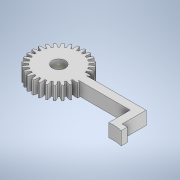
# Autodesk Inventor part: NewConceptArm free V2
Saved by Autodesk Inventor 2022 (Build 260153000, 153)
## iProperties
Created: 2022-02-25
Part Number: NewConceptArm free V2
Material: Generic
Document SubType Name: Modeling
Designer: Alexa
Density: 1 g/cm^3
Appearance: Default
Author: Alexa
Autodesk Inventor part; units mm, degrees
ref_plane "YZ Plane" through (0, 0, 0) normal (1, 0, 0) x (0, 1, 0)
ref_plane "XZ Plane" through (0, 0, 0) normal (0, 1, 0) x (-1, 0, 0)
ref_plane "XY Plane" through (0, 0, 0) normal (0, 0, 1) x (1, 0, 0)
sketch "Sketch1" plane through (0, 0, 0) normal (0, 1, 0) x (-1, 0, 0)
  circle A0 centre (0, 0) radius 8
  circle A1 centre (0, 0) radius 2
  line L0 (7.9113, 0.5933) -> (7.9113, -0.6067)
  line L1 (9.9113, -0.2567) -> (9.9113, 0.2433)
  line L2 (7.6237, -0.0067) -> (9.0479, -0.0067) construction
  arc A2 (9.9113, 0.2433) -> (7.9113, 0.5933) centre (8.1555, -3.9001) ccw construction
  arc A3 (7.9113, -0.6067) -> (9.9113, -0.2567) centre (8.1555, 3.8866) ccw construction
  arc A4 (9.9113, 0.2433) -> (7.9113, 0.5933) centre (8.1555, -3.9001) ccw construction
  arc A5 (9.9113, 0.2433) -> (7.9777, 0.5964) centre (8.1555, -3.9001) ccw
  arc A6 (7.9767, -0.6098) -> (9.9113, -0.2567) centre (8.1555, 3.8866) ccw
  line L3 (9.4, 0) -> (9.4, -0.4379)
  line L4 (9.4, 0) -> (9.4, 0.4244)
  arc A7 (5.296, -1.8919) -> (5.296, 1.8784) centre (4.6281, -0.0067) ccw
  circle A8 centre (0, 0) radius 8
  dimension "d0" = 16
  dimension "d1" = 4
  dimension "d2" = 0.25
  dimension "d3" = 0.25
  dimension "d4" = 0.6
  dimension "d7" = 1.2
  dimension "d8" = 4.5
  dimension "d10" = 2
  constraints: 18 point on circle, 10 end point, 9 centre point, 4 concentric, 3 coincident, 2 vertical, 1 horizontal, 1 parallel, 1 point on line
  measures "d0" diameter of A0
  measures "d1" diameter of A1
  measures "d2" distance from line of L1.start L2
  measures "d3" distance from line of L1.end L2
  measures "d4" distance from line of L0.start L2
  measures "d7" distance of L0.end L0.start
  measures "d8" radius of A3
  measures "d10" radius of A7
extrude "Extrusion1" add sketch "Sketch1" along normal blind 5
pattern_circular "Circular Pattern1" count 28 over 360 about axis through (0, 0, 0) along (0, 1, 0) of "Extrusion1"
sketch "Sketch8" plane through (0, 5, 0) normal (0, 1, 0) x (1, 0, 0)
  circle A0 centre (0, 0) radius 2.5
  circle A1 centre (0, 0) radius 2
  dimension "d49" = 5
  dimension "d50" = 4
  constraints: 2 centre point, 2 coincident
  measures "d49" diameter of A0
  measures "d50" diameter of A1
extrude "Extrusion6" cut sketch "Sketch8" against normal blind 13.8125
sketch "Sketch9" plane through (0, 5, 0) normal (0, 1, 0) x (1, 0, 0)
  circle A0 centre (0, 0) radius 2.5 projected
  line L0 (0, 0) -> (30, 0)
  line L1 (30, 0) -> (30, -18)
  line L2 (30, -18) -> (0, -18)
  line L3 (0, -18) -> (0, 0)
  circle A1 centre (0, 0) radius 9.5
  circle A2 centre (0, -18) radius 9.5
  line L4 (30, -9) -> (0, -9)
  circle A3 centre (30, -9) radius 2.5
  line L5 (30, 0) -> (5, 0)
  line L6 (5, 0) -> (5, -1.5)
  line L7 (5, -1.5) -> (30, -1.5)
  line L8 (30, -1.5) -> (30, 0)
  line L9 (5, 0) -> (30, 0)
  line L10 (30, 0) -> (30, 1.5)
  line L11 (30, 1.5) -> (5, 1.5)
  line L12 (5, 1.5) -> (5, 0)
  line L13 (30, 1.5) -> (31.5, 1.5)
  line L14 (31.5, 1.5) -> (31.5, -7.5)
  line L15 (31.5, -7.5) -> (30, -7.5)
  line L16 (30, -7.5) -> (30, 1.5)
  line L17 (30, 1.5) -> (28.5, 1.5)
  line L18 (28.5, 1.5) -> (28.5, -7.5)
  line L19 (28.5, -7.5) -> (30, -7.5)
  line L20 (30, -7.5) -> (30, 1.5)
  circle A4 centre (30, -9) radius 1.5
  line L21 (27.5, -9) -> (32.5, -9)
  line L22 (32.5, -9) -> (32.5, -8.5)
  line L23 (32.5, -8.5) -> (27.5, -8.5)
  line L24 (27.5, -8.5) -> (27.5, -9)
  line L25 (28.5, -7.5) -> (27.5, -8.5)
  line L26 (31.5, -7.5) -> (32.5, -8.5)
  line L27 (27.5, -8.5) -> (28.5, -8.5)
  line L28 (32.5, -8.5) -> (31.5, -8.5)
  line L29 (28.5, -7.5) -> (29, -7.5)
  line L30 (31.5, -7.5) -> (31, -7.5)
  line L31 (31, -7.5) -> (31.5, -8.5)
  line L32 (29, -7.5) -> (28.5, -8.5)
  line L33 (5, 1.5) -> (12.096, 1.5)
  line L34 (12.096, 1.5) -> (12.096, -1.5)
  line L35 (12.096, -1.5) -> (5, -1.5)
  line L36 (5, -1.5) -> (5, 1.5)
  dimension "d57" = 5
  dimension "d53" = 30
  dimension "d54" = 18
  dimension "d55" = 19
  dimension "d56" = 19
  dimension "d58" = 25
  dimension "d59" = 1.5
  dimension "d60" = 1.5
  dimension "d61" = 1.5
  dimension "d62" = 9
  dimension "d63" = 1.5
  dimension "d64" = 3
  dimension "d65" = 5
  dimension "d66" = 0.5
  dimension "d67" = 0.5
  dimension "d68" = 0.5
  constraints: 74 end point, 14 parallel, 10 point on line, 7 horizontal, 7 perpendicular, 4 coincident, 3 centre point, 2 midpoint, 1 horizontal alignment, 2 other
  measures "d53" distance of L1.end L2.end
  measures "d54" distance of L0.end L1.end
  measures "d55" diameter of A1
  measures "d56" diameter of A2
  measures "d58" distance of L7.end L6.end
  measures "d59" distance of L6.end L5.end
  measures "d60" distance of L10.end L9.end
  measures "d61" distance of L14.end L15.end
  measures "d62" distance of L13.end L14.end
  measures "d63" distance of L19.end L18.end
  measures "d64" diameter of A4
  measures "d65" distance of L23.end L22.end
  measures "d66" distance of L22.end L21.end
  measures "d67" distance of L18.end L29.end
  measures "d68" distance of L14.end L30.end
extrude "Extrusion7" cut sketch "Sketch9" against normal blind 5 contours L12 L11 A1 L0 | L0 A1 L7 L6 | A1 L11 L34 L0 | L0 L34 L7 A1
sketch "Sketch10" plane through (0, 5, 0) normal (0, 1, 0) x (1, 0, 0)
  circle A0 centre (0, 0) radius 2.5 projected
  line L0 (0, 0) -> (30, 0)
  line L1 (30, 0) -> (30, -9)
  line L2 (30, -9) -> (0, -9)
  line L3 (0, -9) -> (0, 0)
  line L4 (5, 1.5) -> (30, 1.5)
  line L5 (30, 1.5) -> (30, -1.5)
  line L6 (30, -1.5) -> (5, -1.5)
  line L7 (5, -1.5) -> (5, 1.5)
  line L8 (31.5, 1.5) -> (28.5, 1.5)
  line L9 (28.5, 1.5) -> (28.5, -7.5)
  line L10 (28.5, -7.5) -> (31.5, -7.5)
  line L11 (31.5, -7.5) -> (31.5, 1.5)
  circle A1 centre (30, -9) radius 1.5
  circle A2 centre (30, -9) radius 2.5
  line L12 (27.5, -9) -> (32.4495, -9)
  line L13 (32.4495, -9) -> (32.4495, -8.5)
  line L14 (27.5, -8.5) -> (27.5, -9)
  line L15 (27.5, -9) -> (32.5, -9)
  line L16 (32.5, -9) -> (32.5, -8.5)
  line L17 (32.5, -8.5) -> (27.5, -8.5)
  line L18 (27.5, -8.5) -> (27.5, -9)
  line L19 (28.5, -7.5) -> (27.5, -8.5)
  line L20 (31.5, -7.5) -> (32.5, -8.5)
  line L21 (28.5, -7.5) -> (29, -7.5)
  line L22 (31.5, -7.5) -> (31, -7.5)
  line L23 (29, -7.5) -> (28.5, -8.5)
  line L24 (31, -7.5) -> (31.5, -8.5)
  point P0 (28.5, -1.5)
  point P1 (28.5, -7)
  point P2 (27.5505, -8.5)
  point P3 (28.5858, -8.5)
  point P4 (31.4142, -8.5)
  point P5 (31.5, -7)
  dimension "d71" = 30
  dimension "d72" = 9
  dimension "d73" = 3
  dimension "d74" = 3
  dimension "d75" = 9
  dimension "d76" = 3
  dimension "d77" = 5
  dimension "d78" = 0.5
  dimension "d79" = 5
  dimension "d80" = 0.5
  dimension "d81" = 0.5
  constraints: 50 end point, 9 parallel, 7 point on line, 6 perpendicular, 5 horizontal, 2 centre point, 2 coincident, 2 point on circle
  measures "d71" distance of L1.end L2.end
  measures "d72" distance of L0.end L1.end
  measures "d73" distance of L4.end L5.end
  measures "d74" distance of L10.end L9.end
  measures "d75" distance of L9.end L8.end
  measures "d76" diameter of A1
  measures "d77" diameter of A2
  measures "d78" distance of L13.end L12.end
  measures "d79" distance of L17.end L16.end
  measures "d80" distance of L9.end L21.end
  measures "d81" distance of L10.end L22.end
extrude "Extrusion8" add sketch "Sketch10" against normal blind 5 contours L7 L4 L9 L0 | L0 L9 L6 L7 | L9 L4 L5 L0 | L0 L1 L6 L9 | L5 L8 L11 A2 L1 | L6 L1 A2 L9 | A2 L19 L10 L23 L17 | A2 L1 L10 L9 | L9 L19 A2 | L17 L23 L10 A1 | L17 L24 L10 L20 A2 | A2 L11 L10 L1 | L10 L24 L17 A1 | L20 L11 A2
sketch "Sketch11" plane through (0, 5, 0) normal (0, 1, 0) x (1, 0, 0)
  arc A0 (31.4142, -8.5) -> (28.5858, -8.5) centre (30, -9) ccw projected
  circle A1 centre (30, -9) radius 1.5
  line L0 (30, 0) -> (30, -9)
  line L1 (33.5287, -9.8898) -> (25.3685, -9.8898)
  line L2 (25.3685, -9.8898) -> (25.3685, -3.9183)
  line L3 (25.3685, -3.9183) -> (33.5287, -3.9183)
  line L4 (33.5287, -3.9183) -> (33.5287, -9.8898)
  point P0 (0, 0)
  point P1 (28.7925, -9.8898)
  point P2 (31.2075, -9.8898)
  constraints: 10 end point, 2 parallel, 1 centre point, 1 coincident, 1 horizontal, 1 perpendicular, 1 vertical
extrude "Extrusion9" cut sketch "Sketch11" against normal blind 7.4625 contours A0 L0 L3 L4 L1 A1 | A0 A1 L1 L2 L3 L0
sketch "Sketch14" plane through (0, 5, 0) normal (0, 1, 0) x (1, 0, 0)
  line L0 (0, 0) -> (30, 0)
  line L1 (30, 0) -> (30, -10)
  line L2 (30, -10) -> (0, -10)
  line L3 (0, -10) -> (0, 0)
  line L4 (30, 0) -> (30, -25)
  circle A0 centre (30, -25) radius 15.5
  line L5 (31.5, -3.9183) -> (31.5, 1.5) projected
  line L6 (31.5, 0) -> (22.5, 0)
  line L7 (22.5, 0) -> (22.5, -9.2288)
  line L8 (22.5, -9.2288) -> (31.5, -9.2288)
  line L9 (31.5, -9.2288) -> (31.5, 0)
  line L10 (31.5, -3.9183) -> (28.5, -3.9183) projected
  line L11 (31.5, -3.9183) -> (28.5, -3.9183)
  line L12 (28.5, -3.9183) -> (28.5, -9.2288)
  line L13 (28.5, -9.2288) -> (31.5, -9.2288)
  line L14 (31.5, -9.2288) -> (31.5, -3.9183)
  line L15 (31.5, 0) -> (31.5, -9.5728)
  line L16 (28.5, -3.9183) -> (28.5, -1.5) projected
  line L17 (28.5, -1.5) -> (28.5, -9.5728)
  line L18 (31.5, -9.5728) -> (34.5, -9.5728)
  line L19 (28.5, -3.9183) -> (31.5, -3.9183) projected
  line L20 (28.5, -9.5728) -> (25.5, -9.5728)
  line L21 (25.5, -9.5728) -> (25.5, -10.1676)
  line L22 (34.5, -9.5728) -> (34.5, -10.1676)
  line L23 (34.5, -9.5728) -> (31.5, -9.5728)
  line L24 (31.5, -9.5728) -> (31.5, -7.5728)
  line L25 (31.5, -7.5728) -> (34.5, -7.5728)
  line L26 (34.5, -7.5728) -> (34.5, -9.5728)
  line L27 (28.5, -9.5728) -> (25.5, -9.5728)
  line L28 (25.5, -9.5728) -> (25.5, -7.5728)
  line L29 (25.5, -7.5728) -> (28.5, -7.5728)
  line L30 (28.5, -7.5728) -> (28.5, -9.5728)
  point P0 (25.5, -10)
  point P1 (26.0949, -10)
  dimension "d93" = 30
  dimension "d94" = 10
  dimension "d95" = 25
  dimension "d96" = 31
  dimension "d97" = 9
  dimension "d98" = 3
  dimension "d99" = 3
  dimension "d100" = 2
  dimension "d101" = 3
  dimension "d102" = 2
  constraints: 54 end point, 12 parallel, 6 perpendicular, 6 point on line, 5 horizontal, 4 point on circle, 1 centre point, 1 coincident
  measures "d93" distance of L1.end L2.end
  measures "d94" distance of L0.end L1.end
  measures "d95" distance of L0.end L4.end
  measures "d96" diameter of A0
  measures "d97" distance of L8.end L7.end
  measures "d98" distance of L15.end L18.end
  measures "d99" distance of L17.end L20.end
  measures "d100" distance of L23.end L24.end
  measures "d101" distance of L28.end L29.end
  measures "d102" distance of L27.end L28.end
extrude "Extrusion10" add sketch "Sketch14" against normal blind 5 contours L21 L20 A0 L2 | L10 L9 L8 L1 | L1 L8 L12 L10 | L28 L29 L12 L8 | L8 L17 L20 L28 | L8 L15 A0 L1 | L1 A0 L17 L8 | L9 L25 L26 L18 L15 | A0 L18 L22
sketch "Sketch15" plane through (0, 5, 0) normal (0, 1, 0) x (1, 0, 0)
  line L0 (25.5, -7.5728) -> (28.5, -7.5728) projected
  line L1 (25.5, -7.5728) -> (27.5, -7.5728)
  line L2 (27.5, -7.5728) -> (27.5, -11.2881)
  line L3 (27.5, -11.2881) -> (25.5, -11.2881)
  line L4 (25.5, -11.2881) -> (25.5, -7.5728)
  line L5 (31.5, -7.5728) -> (34.5, -7.5728) projected
  line L6 (34.5, -7.5728) -> (32.5, -7.5728)
  line L7 (32.5, -7.5728) -> (32.5, -12.173)
  line L8 (32.5, -12.173) -> (34.5, -12.173)
  line L9 (34.5, -12.173) -> (34.5, -7.5728)
  line L10 (34.5, -7.5728) -> (33.5, -7.5728)
  line L11 (33.5, -7.5728) -> (33.5, -13.7619)
  line L12 (33.5, -13.7619) -> (34.5, -13.7619)
  line L13 (34.5, -13.7619) -> (34.5, -7.5728)
  point P0 (0, 0)
  point P1 (33.5, -12.173)
  dimension "d105" = 2
  dimension "d106" = 2
  constraints: 24 end point, 6 parallel, 3 horizontal, 3 perpendicular
  measures "d105" distance of L2.end L3.end
  measures "d106" distance of L8.end L7.end
extrude "Extrusion11" cut sketch "Sketch15" against normal blind 7.7 contours L0 L2 L3 L4 | L5 L9 L8 L11
sketch "Sketch16" plane through (0, 5, 0) normal (0, 1, 0) x (1, 0, 0)
  line L0 (27.5, -9.7029) -> (27.5, -7.5728) projected
  line L1 (27.5, -7.5728) -> (28.5, -7.5728)
  line L2 (28.5, -7.5728) -> (28.5, -10.975)
  line L3 (28.5, -10.975) -> (27.5, -10.975)
  line L4 (27.5, -10.975) -> (27.5, -7.5728)
  point P0 (0, 0)
  dimension "d109" = 1
  constraints: 8 end point, 2 parallel, 1 horizontal, 1 perpendicular
  measures "d109" distance of L2.end L3.end
extrude "Extrusion12" cut sketch "Sketch16" against normal blind 12.9375
sketch "Sketch17" plane through (0, 5, 0) normal (0, 1, 0) x (1, 0, 0)
  point P0 (0, 0)
body "Solid1"
